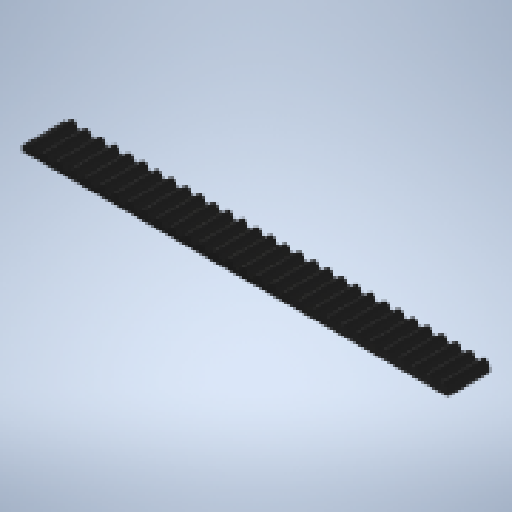
# Autodesk Inventor part: GT2BeltSegment
Saved by Autodesk Inventor 2023 (Build 270158000, 158)
## iProperties
Created: 2023-08-18
Part Number: GT2BeltSegment
Material: Generic
Document SubType Name: Modeling
Designer: Felix
Density: 1 g/cm^3
Appearance: Smooth - Black
Author: Felix
Autodesk Inventor part; units mm, degrees
ref_plane "YZ Plane" through (0, 0, 0) normal (1, 0, 0) x (0, 1, 0)
ref_plane "XZ Plane" through (0, 0, 0) normal (0, 1, 0) x (-1, 0, 0)
ref_plane "XY Plane" through (0, 0, 0) normal (0, 0, 1) x (1, 0, 0)
sketch "Sketch1" plane through (0, 0, 0) normal (0, 0, 1) x (1, 0, 0)
  line L0 (0, 0) -> (5.6329, 0)
  line L1 (0, 0.376) -> (6.7417, 0.376) construction
  line L2 (0, 0.63) -> (0.5196, 0.63)
  line L3 (1.2598, 0) -> (1.2598, 2.5945) construction
  arc A0 (0.5196, 0.63) -> (0.6684, 0.7604) centre (0.5196, 0.78) ccw
  arc A1 (0.7709, 1.0881) -> (0.6684, 0.7604) centre (1.6598, 0.63) ccw
  arc A2 (1.7487, 1.0881) -> (0.7709, 1.0881) centre (1.2598, 0.8362) ccw
  arc A3 (1.8513, 0.7604) -> (2, 0.63) centre (2, 0.78) ccw
  arc A4 (1.8513, 0.7604) -> (1.7487, 1.0881) centre (0.8598, 0.63) ccw
  line L4 (0, 0.63) -> (0, 0)
  line L5 (2, 0.63) -> (2.5196, 0.63)
  arc A5 (2.5196, 0.63) -> (2.6684, 0.7604) centre (2.5196, 0.78) ccw
  arc A6 (2.7709, 1.0881) -> (2.6684, 0.7604) centre (3.6598, 0.63) ccw
  arc A7 (3.8513, 0.7604) -> (3.7487, 1.0881) centre (2.8598, 0.63) ccw
  arc A8 (3.7487, 1.0881) -> (2.7709, 1.0881) centre (3.2598, 0.8362) ccw
  arc A9 (3.8513, 0.7604) -> (4, 0.63) centre (4, 0.78) ccw
  line L6 (4, 0.63) -> (4.5196, 0.63)
  arc A10 (4.5196, 0.63) -> (4.6684, 0.7604) centre (4.5196, 0.78) ccw
  arc A11 (4.7709, 1.0881) -> (4.6684, 0.7604) centre (5.6598, 0.63) ccw
  arc A12 (5.8513, 0.7604) -> (5.7487, 1.0881) centre (4.8598, 0.63) ccw
  arc A13 (5.7487, 1.0881) -> (4.7709, 1.0881) centre (5.2598, 0.8362) ccw
  arc A14 (5.8513, 0.7604) -> (6, 0.63) centre (6, 0.78) ccw
  line L7 (6, 0.63) -> (6.5196, 0.63)
  arc A15 (6.5196, 0.63) -> (6.6684, 0.7604) centre (6.5196, 0.78) ccw
  arc A16 (6.7709, 1.0881) -> (6.6684, 0.7604) centre (7.6598, 0.63) ccw
  arc A17 (7.8513, 0.7604) -> (7.7487, 1.0881) centre (6.8598, 0.63) ccw
  arc A18 (7.7487, 1.0881) -> (6.7709, 1.0881) centre (7.2598, 0.8362) ccw
  arc A19 (7.8513, 0.7604) -> (8, 0.63) centre (8, 0.78) ccw
  line L8 (8, 0.63) -> (8.5196, 0.63)
  arc A20 (8.5196, 0.63) -> (8.6684, 0.7604) centre (8.5196, 0.78) ccw
  arc A21 (8.7709, 1.0881) -> (8.6684, 0.7604) centre (9.6598, 0.63) ccw
  arc A22 (9.8513, 0.7604) -> (9.7487, 1.0881) centre (8.8598, 0.63) ccw
  arc A23 (9.7487, 1.0881) -> (8.7709, 1.0881) centre (9.2598, 0.8362) ccw
  arc A24 (9.8513, 0.7604) -> (10, 0.63) centre (10, 0.78) ccw
  line L9 (10, 0.63) -> (10.5196, 0.63)
  arc A25 (10.5196, 0.63) -> (10.6684, 0.7604) centre (10.5196, 0.78) ccw
  arc A26 (10.7709, 1.0881) -> (10.6684, 0.7604) centre (11.6598, 0.63) ccw
  arc A27 (11.8513, 0.7604) -> (11.7487, 1.0881) centre (10.8598, 0.63) ccw
  arc A28 (11.7487, 1.0881) -> (10.7709, 1.0881) centre (11.2598, 0.8362) ccw
  arc A29 (11.8513, 0.7604) -> (12, 0.63) centre (12, 0.78) ccw
  line L10 (12, 0.63) -> (12.5196, 0.63)
  arc A30 (12.5196, 0.63) -> (12.6684, 0.7604) centre (12.5196, 0.78) ccw
  arc A31 (12.7709, 1.0881) -> (12.6684, 0.7604) centre (13.6598, 0.63) ccw
  arc A32 (13.8513, 0.7604) -> (13.7487, 1.0881) centre (12.8598, 0.63) ccw
  arc A33 (13.7487, 1.0881) -> (12.7709, 1.0881) centre (13.2598, 0.8362) ccw
  arc A34 (13.8513, 0.7604) -> (14, 0.63) centre (14, 0.78) ccw
  line L11 (14, 0.63) -> (14.5196, 0.63)
  arc A35 (14.5196, 0.63) -> (14.6684, 0.7604) centre (14.5196, 0.78) ccw
  arc A36 (14.7709, 1.0881) -> (14.6684, 0.7604) centre (15.6598, 0.63) ccw
  arc A37 (15.8513, 0.7604) -> (15.7487, 1.0881) centre (14.8598, 0.63) ccw
  arc A38 (15.7487, 1.0881) -> (14.7709, 1.0881) centre (15.2598, 0.8362) ccw
  arc A39 (15.8513, 0.7604) -> (16, 0.63) centre (16, 0.78) ccw
  line L12 (16, 0.63) -> (16.5196, 0.63)
  arc A40 (16.5196, 0.63) -> (16.6684, 0.7604) centre (16.5196, 0.78) ccw
  arc A41 (16.7709, 1.0881) -> (16.6684, 0.7604) centre (17.6598, 0.63) ccw
  arc A42 (17.8513, 0.7604) -> (17.7487, 1.0881) centre (16.8598, 0.63) ccw
  arc A43 (17.7487, 1.0881) -> (16.7709, 1.0881) centre (17.2598, 0.8362) ccw
  arc A44 (17.8513, 0.7604) -> (18, 0.63) centre (18, 0.78) ccw
  line L13 (18, 0.63) -> (18.5196, 0.63)
  arc A45 (18.5196, 0.63) -> (18.6684, 0.7604) centre (18.5196, 0.78) ccw
  arc A46 (18.7709, 1.0881) -> (18.6684, 0.7604) centre (19.6598, 0.63) ccw
  arc A47 (19.8513, 0.7604) -> (19.7487, 1.0881) centre (18.8598, 0.63) ccw
  arc A48 (19.7487, 1.0881) -> (18.7709, 1.0881) centre (19.2598, 0.8362) ccw
  arc A49 (19.8513, 0.7604) -> (20, 0.63) centre (20, 0.78) ccw
  line L14 (20, 0.63) -> (20.5196, 0.63)
  arc A50 (20.5196, 0.63) -> (20.6684, 0.7604) centre (20.5196, 0.78) ccw
  arc A51 (20.7709, 1.0881) -> (20.6684, 0.7604) centre (21.6598, 0.63) ccw
  arc A52 (21.8513, 0.7604) -> (21.7487, 1.0881) centre (20.8598, 0.63) ccw
  arc A53 (21.7487, 1.0881) -> (20.7709, 1.0881) centre (21.2598, 0.8362) ccw
  arc A54 (21.8513, 0.7604) -> (22, 0.63) centre (22, 0.78) ccw
  line L15 (22, 0.63) -> (22.5196, 0.63)
  arc A55 (22.5196, 0.63) -> (22.6684, 0.7604) centre (22.5196, 0.78) ccw
  arc A56 (22.7709, 1.0881) -> (22.6684, 0.7604) centre (23.6598, 0.63) ccw
  arc A57 (23.8513, 0.7604) -> (23.7487, 1.0881) centre (22.8598, 0.63) ccw
  arc A58 (23.7487, 1.0881) -> (22.7709, 1.0881) centre (23.2598, 0.8362) ccw
  arc A59 (23.8513, 0.7604) -> (24, 0.63) centre (24, 0.78) ccw
  line L16 (24, 0.63) -> (24.5196, 0.63)
  arc A60 (24.5196, 0.63) -> (24.6684, 0.7604) centre (24.5196, 0.78) ccw
  arc A61 (24.7709, 1.0881) -> (24.6684, 0.7604) centre (25.6598, 0.63) ccw
  arc A62 (25.8513, 0.7604) -> (25.7487, 1.0881) centre (24.8598, 0.63) ccw
  arc A63 (25.7487, 1.0881) -> (24.7709, 1.0881) centre (25.2598, 0.8362) ccw
  arc A64 (25.8513, 0.7604) -> (26, 0.63) centre (26, 0.78) ccw
  line L17 (26, 0.63) -> (26.5196, 0.63)
  arc A65 (26.5196, 0.63) -> (26.6684, 0.7604) centre (26.5196, 0.78) ccw
  arc A66 (26.7709, 1.0881) -> (26.6684, 0.7604) centre (27.6598, 0.63) ccw
  arc A67 (27.8513, 0.7604) -> (27.7487, 1.0881) centre (26.8598, 0.63) ccw
  arc A68 (27.7487, 1.0881) -> (26.7709, 1.0881) centre (27.2598, 0.8362) ccw
  arc A69 (27.8513, 0.7604) -> (28, 0.63) centre (28, 0.78) ccw
  line L18 (28, 0.63) -> (28.5196, 0.63)
  arc A70 (28.5196, 0.63) -> (28.6684, 0.7604) centre (28.5196, 0.78) ccw
  arc A71 (28.7709, 1.0881) -> (28.6684, 0.7604) centre (29.6598, 0.63) ccw
  arc A72 (29.8513, 0.7604) -> (29.7487, 1.0881) centre (28.8598, 0.63) ccw
  arc A73 (29.7487, 1.0881) -> (28.7709, 1.0881) centre (29.2598, 0.8362) ccw
  arc A74 (29.8513, 0.7604) -> (30, 0.63) centre (30, 0.78) ccw
  line L19 (30, 0.63) -> (30.5196, 0.63)
  arc A75 (30.5196, 0.63) -> (30.6684, 0.7604) centre (30.5196, 0.78) ccw
  arc A76 (30.7709, 1.0881) -> (30.6684, 0.7604) centre (31.6598, 0.63) ccw
  arc A77 (31.8513, 0.7604) -> (31.7487, 1.0881) centre (30.8598, 0.63) ccw
  arc A78 (31.7487, 1.0881) -> (30.7709, 1.0881) centre (31.2598, 0.8362) ccw
  arc A79 (31.8513, 0.7604) -> (32, 0.63) centre (32, 0.78) ccw
  line L20 (32, 0.63) -> (32.5196, 0.63)
  arc A80 (32.5196, 0.63) -> (32.6684, 0.7604) centre (32.5196, 0.78) ccw
  arc A81 (32.7709, 1.0881) -> (32.6684, 0.7604) centre (33.6598, 0.63) ccw
  arc A82 (33.8513, 0.7604) -> (33.7487, 1.0881) centre (32.8598, 0.63) ccw
  arc A83 (33.7487, 1.0881) -> (32.7709, 1.0881) centre (33.2598, 0.8362) ccw
  arc A84 (33.8513, 0.7604) -> (34, 0.63) centre (34, 0.78) ccw
  line L21 (34, 0.63) -> (34.5196, 0.63)
  arc A85 (34.5196, 0.63) -> (34.6684, 0.7604) centre (34.5196, 0.78) ccw
  arc A86 (34.7709, 1.0881) -> (34.6684, 0.7604) centre (35.6598, 0.63) ccw
  arc A87 (35.8513, 0.7604) -> (35.7487, 1.0881) centre (34.8598, 0.63) ccw
  arc A88 (35.7487, 1.0881) -> (34.7709, 1.0881) centre (35.2598, 0.8362) ccw
  arc A89 (35.8513, 0.7604) -> (36, 0.63) centre (36, 0.78) ccw
  line L22 (36, 0.63) -> (36.5196, 0.63)
  arc A90 (36.5196, 0.63) -> (36.6684, 0.7604) centre (36.5196, 0.78) ccw
  arc A91 (36.7709, 1.0881) -> (36.6684, 0.7604) centre (37.6598, 0.63) ccw
  arc A92 (37.8513, 0.7604) -> (37.7487, 1.0881) centre (36.8598, 0.63) ccw
  arc A93 (37.7487, 1.0881) -> (36.7709, 1.0881) centre (37.2598, 0.8362) ccw
  arc A94 (37.8513, 0.7604) -> (38, 0.63) centre (38, 0.78) ccw
  line L23 (38, 0.63) -> (38.5196, 0.63)
  arc A95 (38.5196, 0.63) -> (38.6684, 0.7604) centre (38.5196, 0.78) ccw
  arc A96 (38.7709, 1.0881) -> (38.6684, 0.7604) centre (39.6598, 0.63) ccw
  arc A97 (39.8513, 0.7604) -> (39.7487, 1.0881) centre (38.8598, 0.63) ccw
  arc A98 (39.7487, 1.0881) -> (38.7709, 1.0881) centre (39.2598, 0.8362) ccw
  arc A99 (39.8513, 0.7604) -> (40, 0.63) centre (40, 0.78) ccw
  line L24 (40, 0.63) -> (40.5196, 0.63)
  arc A100 (40.5196, 0.63) -> (40.6684, 0.7604) centre (40.5196, 0.78) ccw
  arc A101 (40.7709, 1.0881) -> (40.6684, 0.7604) centre (41.6598, 0.63) ccw
  arc A102 (41.8513, 0.7604) -> (41.7487, 1.0881) centre (40.8598, 0.63) ccw
  arc A103 (41.7487, 1.0881) -> (40.7709, 1.0881) centre (41.2598, 0.8362) ccw
  arc A104 (41.8513, 0.7604) -> (42, 0.63) centre (42, 0.78) ccw
  line L25 (42, 0.63) -> (42.5196, 0.63)
  arc A105 (42.5196, 0.63) -> (42.6684, 0.7604) centre (42.5196, 0.78) ccw
  arc A106 (42.7709, 1.0881) -> (42.6684, 0.7604) centre (43.6598, 0.63) ccw
  arc A107 (43.8513, 0.7604) -> (43.7487, 1.0881) centre (42.8598, 0.63) ccw
  arc A108 (43.7487, 1.0881) -> (42.7709, 1.0881) centre (43.2598, 0.8362) ccw
  arc A109 (43.8513, 0.7604) -> (44, 0.63) centre (44, 0.78) ccw
  line L26 (44, 0.63) -> (44.5196, 0.63)
  arc A110 (44.5196, 0.63) -> (44.6684, 0.7604) centre (44.5196, 0.78) ccw
  arc A111 (44.7709, 1.0881) -> (44.6684, 0.7604) centre (45.6598, 0.63) ccw
  arc A112 (45.8513, 0.7604) -> (45.7487, 1.0881) centre (44.8598, 0.63) ccw
  arc A113 (45.7487, 1.0881) -> (44.7709, 1.0881) centre (45.2598, 0.8362) ccw
  arc A114 (45.8513, 0.7604) -> (46, 0.63) centre (46, 0.78) ccw
  line L27 (46, 0.63) -> (46.5196, 0.63)
  arc A115 (46.5196, 0.63) -> (46.6684, 0.7604) centre (46.5196, 0.78) ccw
  arc A116 (46.7709, 1.0881) -> (46.6684, 0.7604) centre (47.6598, 0.63) ccw
  arc A117 (47.8513, 0.7604) -> (47.7487, 1.0881) centre (46.8598, 0.63) ccw
  arc A118 (47.7487, 1.0881) -> (46.7709, 1.0881) centre (47.2598, 0.8362) ccw
  arc A119 (47.8513, 0.7604) -> (48, 0.63) centre (48, 0.78) ccw
  line L28 (48, 0.63) -> (48.5196, 0.63)
  arc A120 (48.5196, 0.63) -> (48.6684, 0.7604) centre (48.5196, 0.78) ccw
  arc A121 (48.7709, 1.0881) -> (48.6684, 0.7604) centre (49.6598, 0.63) ccw
  arc A122 (49.8513, 0.7604) -> (49.7487, 1.0881) centre (48.8598, 0.63) ccw
  arc A123 (49.7487, 1.0881) -> (48.7709, 1.0881) centre (49.2598, 0.8362) ccw
  arc A124 (49.8513, 0.7604) -> (50, 0.63) centre (50, 0.78) ccw
  line L29 (50, 0.63) -> (50.5196, 0.63)
  arc A125 (50.5196, 0.63) -> (50.6684, 0.7604) centre (50.5196, 0.78) ccw
  arc A126 (50.7709, 1.0881) -> (50.6684, 0.7604) centre (51.6598, 0.63) ccw
  arc A127 (51.8513, 0.7604) -> (51.7487, 1.0881) centre (50.8598, 0.63) ccw
  arc A128 (51.7487, 1.0881) -> (50.7709, 1.0881) centre (51.2598, 0.8362) ccw
  arc A129 (51.8513, 0.7604) -> (52, 0.63) centre (52, 0.78) ccw
  line L30 (52, 0.63) -> (52.5196, 0.63)
  arc A130 (52.5196, 0.63) -> (52.6684, 0.7604) centre (52.5196, 0.78) ccw
  arc A131 (52.7709, 1.0881) -> (52.6684, 0.7604) centre (53.6598, 0.63) ccw
  arc A132 (53.8513, 0.7604) -> (53.7487, 1.0881) centre (52.8598, 0.63) ccw
  arc A133 (53.7487, 1.0881) -> (52.7709, 1.0881) centre (53.2598, 0.8362) ccw
  arc A134 (53.8513, 0.7604) -> (54, 0.63) centre (54, 0.78) ccw
  line L31 (54, 0.63) -> (54.5196, 0.63)
  arc A135 (54.5196, 0.63) -> (54.6684, 0.7604) centre (54.5196, 0.78) ccw
  arc A136 (54.7709, 1.0881) -> (54.6684, 0.7604) centre (55.6598, 0.63) ccw
  arc A137 (55.8513, 0.7604) -> (55.7487, 1.0881) centre (54.8598, 0.63) ccw
  arc A138 (55.7487, 1.0881) -> (54.7709, 1.0881) centre (55.2598, 0.8362) ccw
  arc A139 (55.8513, 0.7604) -> (56, 0.63) centre (56, 0.78) ccw
  line L32 (56, 0.63) -> (56.5196, 0.63)
  arc A140 (56.5196, 0.63) -> (56.6684, 0.7604) centre (56.5196, 0.78) ccw
  arc A141 (56.7709, 1.0881) -> (56.6684, 0.7604) centre (57.6598, 0.63) ccw
  arc A142 (57.8513, 0.7604) -> (57.7487, 1.0881) centre (56.8598, 0.63) ccw
  arc A143 (57.7487, 1.0881) -> (56.7709, 1.0881) centre (57.2598, 0.8362) ccw
  arc A144 (57.8513, 0.7604) -> (58, 0.63) centre (58, 0.78) ccw
  line L33 (58, 0.63) -> (58.5196, 0.63)
  arc A145 (58.5196, 0.63) -> (58.6684, 0.7604) centre (58.5196, 0.78) ccw
  arc A146 (58.7709, 1.0881) -> (58.6684, 0.7604) centre (59.6598, 0.63) ccw
  arc A147 (59.8513, 0.7604) -> (59.7487, 1.0881) centre (58.8598, 0.63) ccw
  arc A148 (59.7487, 1.0881) -> (58.7709, 1.0881) centre (59.2598, 0.8362) ccw
  arc A149 (59.8513, 0.7604) -> (60, 0.63) centre (60, 0.78) ccw
  line L34 (60, 0.63) -> (60, 0)
  line L35 (60, 0) -> (0, 0)
  point P0 (50, 0.63)
  point P1 (36, 0.63)
  point P2 (30, 0.63)
  point P3 (26, 0.63)
  point P4 (18, 0.63)
  point P5 (14, 0.63)
  point P6 (12, 0.63)
  dimension "d0" = 0.376
  dimension "d1" = 0.254
  dimension "d2" = 0.15
  dimension "d3" = 1
  dimension "d4" = 0.4
  dimension "d6" = 0.55
  dimension "d7" = 2
  dimension "d10" = 2
  constraints: 300 point on circle, 150 centre point, 72 end point, 5 symmetric about line, 4 horizontal, 3 tangent, 3 vertical, 1 horizontal alignment, 1 perpendicular, 1 point on line, 1 vertical alignment, 524 other
  measures "d0" distance between parallel lines of L0 L1
  measures "d1" distance between parallel lines of L1 L2
  measures "d2" radius of A0
  measures "d3" radius of A1
  measures "d4" distance from line of L3 A1.centre
  measures "d6" radius of A2
  measures "d7" distance of A3.end L2.start
  measures "d10" distance of L2.end L5.end
extrude "Extrusion1" add sketch "Sketch1" along normal blind 6
body "Solid1"
